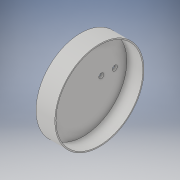
# Autodesk Inventor part: Top Sensor Base v1.2
Saved by Autodesk Inventor 2019 (Build 230136000, 136)
## iProperties
Created: 2020-01-12
Part Number: Top Sensor Base v1.2
Material: Generic
Document SubType Name: Modeling
Designer: Obscure_Decision
Density: 1 g/cm^3
Appearance: Default
Author: Obscure_Decision
Autodesk Inventor part; units mm, degrees
ref_plane "YZ Plane" through (0, 0, 0) normal (1, 0, 0) x (0, 1, 0)
ref_plane "XZ Plane" through (0, 0, 0) normal (0, 1, 0) x (-1, 0, 0)
ref_plane "XY Plane" through (0, 0, 0) normal (0, 0, 1) x (1, 0, 0)
sketch "Sketch1" plane through (0, 0, 0) normal (0, 1, 0) x (-1, 0, 0)
  line L0 (0, 0) -> (3.0988, 0)
  line L1 (3.0988, 0) -> (3.0988, -47.498)
  line L2 (3.0988, -47.498) -> (0, -47.498)
  line L3 (0, -47.498) -> (0, 0)
  line L4 (3.0988, 0) -> (0, 0)
  line L5 (0, 0) -> (0, -49.53)
  line L6 (0, -49.53) -> (3.0988, -49.53)
  line L7 (3.0988, -49.53) -> (3.0988, 0)
  dimension "d0" = 3.0988
  dimension "d1" = 47.498
  dimension "d2" = 49.53
  constraints: 16 end point, 4 parallel, 2 horizontal, 2 perpendicular
  measures "d0" distance of L1.end L2.end
  measures "d1" distance of L0.end L1.end
  measures "d2" distance of L4.end L5.end
revolve "top base" add sketch "Sketch1" angle 360 about axis through (-3.0988, 0, 0) along (1, 0, 0)
sketch "outer wall" plane through (0, 0, 0) normal (1, 0, 0) x (0, 0, -1)
  circle A0 centre (0, 0) radius 48.26
  circle A1 centre (0, 0) radius 49.53
  dimension "d4" = 96.52
  dimension "d7" = 99.06
  constraints: 2 centre point, 2 coincident
  measures "d4" diameter of A0
  measures "d7" diameter of A1
extrude "top outer wall" add sketch "outer wall" along normal blind 17.78
sketch "top circles" plane through (0, 0, 0) normal (1, 0, 0) x (0, 0, -1)
  line L0 (27.4022, -6.3354) -> (27.4022, 6.3646) construction
  circle A0 centre (34.8952, 0.0146) radius 2.794
  circle A1 centre (19.9092, 0.0146) radius 2.794
  line L1 (22.7032, 0.0146) -> (32.1012, 0.0146) construction
  line L2 (14.7022, -6.3354) -> (40.1022, -6.3354) construction
  line L3 (40.1022, -6.3354) -> (40.1022, 6.3646) construction
  line L4 (40.1022, 6.3646) -> (14.7022, 6.3646) construction
  line L5 (14.7022, 6.3646) -> (14.7022, -6.3354) construction
  line L6 (14.7022, -6.3354) -> (40.1022, 6.3646) construction
  line L7 (40.1022, -6.3354) -> (14.7022, 6.3646) construction
  line L8 (40.065, -6.3646) -> (-40.065, -6.3646)
  line L9 (-40.065, -6.3646) -> (-40.065, 6.3646)
  line L10 (-40.065, 6.3646) -> (40.065, 6.3646)
  line L11 (40.065, 6.3646) -> (40.065, -6.3646)
  line L12 (40.065, -6.3646) -> (-40.065, 6.3646) construction
  line L13 (-40.065, -6.3646) -> (40.065, 6.3646) construction
  circle A2 centre (0, 0) radius 48.26 projected
  point P0 (27.4022, 0.0146)
  dimension "d30" = 9.398
  dimension "d31" = 8.001
  dimension "d32" = 8.001
  dimension "d33" = 80.13
  constraints: 28 end point, 5 midpoint, 4 parallel, 3 horizontal, 2 horizontal alignment, 2 perpendicular, 1 symmetric about line, 1 vertical, 4 other
  measures "d30" distance of L1.start L1.end
  measures "d31" distance from line of L5 L1.start
  measures "d32" distance from line of L3 L1.end
  measures "d33" distance of L9.end L10.end
extrude "Top holes" cut sketch "top circles" against normal blind 25.4 contours A0 | A1
body "Solid1"
